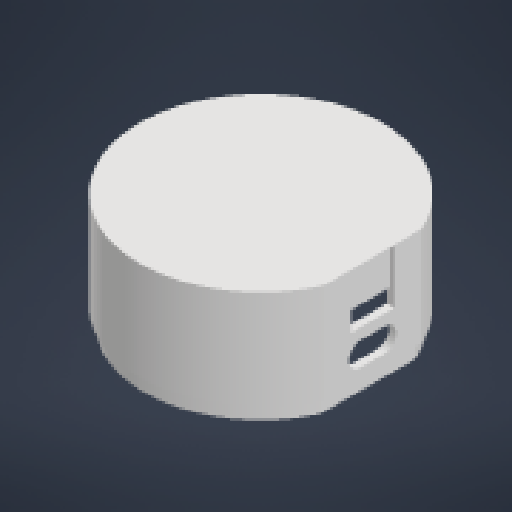
# Autodesk Inventor part: Boden
Saved by Autodesk Inventor 2026 (Build 300175000, 175)
## iProperties
Created: 2025-04-23
Part Number: Boden
Material: Generisch
Document SubType Name: Modeling
Designer: HTL
Density: 1 g/cm^3
Appearance: Vorgabe
Author: HTL
Autodesk Inventor part; units mm, degrees
ref_plane "YZ Plane" through (0, 0, 0) normal (1, 0, 0) x (0, 1, 0)
ref_plane "XZ Plane" through (0, 0, 0) normal (0, 1, 0) x (-1, 0, 0)
ref_plane "XY Plane" through (0, 0, 0) normal (0, 0, 1) x (1, 0, 0)
ref_plane "Arbeitsebene1" through (16.6353, -6.4369, 0) normal (0, 0, 1) x (1, 0, 0)
sketch "Skizze1" plane through (16.6353, -6.4369, 0) normal (0, 0, 1) x (1, 0, 0)
  circle A0 centre (-16.6375, -8.7) radius 1.3
  circle A1 centre (-16.6375, 8.7) radius 1.3
  circle A2 centre (23.3088, -8.7) radius 1.3
  circle A3 centre (23.3715, 8.7) radius 1.3
  point P0 (-16.6353, 6.4369)
  constraints: 4 centre point
extrude "Extrusion1" add sketch "Skizze1" along normal mid plane 4
ref_plane "Arbeitsebene3" through (16.6353, -6.4369, 0) normal (0, 0, 1) x (1, 0, 0)
sketch "Skizze11" plane through (16.6353, -6.4369, 0) normal (0, 0, 1) x (1, 0, 0)
  line L0 (19.6375, -11.7) -> (-19.6375, -11.7)
  line L1 (-19.6375, -11.7) -> (-19.6375, 11.7)
  line L2 (-20.6375, 12.7) -> (27.3715, 12.7)
  line L3 (-19.6375, 11.7) -> (-19.6375, -11.7)
  line L4 (-19.6375, -11.7) -> (26.3715, -11.7)
  line L5 (26.3715, -11.7) -> (26.3715, 11.7)
  line L6 (-19.6375, 11.7) -> (26.3715, 11.7)
  line L7 (-20.6375, -12.7) -> (27.3715, -12.7)
  line L8 (27.3715, -12.7) -> (27.3715, 12.7)
  line L9 (-20.6375, -12.7) -> (27.3715, -12.7)
  line L10 (27.3715, -12.7) -> (27.3715, 12.7)
  line L11 (27.3715, 12.7) -> (-20.6375, 12.7)
  line L12 (-20.6375, 12.7) -> (-20.6375, -12.7)
  point P0 (-16.6353, 6.4369)
  point P1 (19.6375, -11.7)
  constraints: 26 end point, 3 horizontal, 3 parallel, 3 perpendicular
sketch "Skizze12" plane through (16.6353, -6.4369, 2) normal (0, 0, 1) x (1, 0, 0)
  line L0 (20.6375, 12.7) -> (-20.6375, 12.7) projected
  line L1 (-20.6375, 12.7) -> (-20.6375, -12.7) projected
  line L2 (-20.6375, -12.7) -> (20.6375, -12.7) projected
  line L3 (20.6375, -12.7) -> (20.6375, 12.7) projected
  circle A0 centre (0, 0) radius 32
  line L4 (20.6375, 12.7) -> (29.3719, 12.7)
  line L5 (29.3719, -12.7) -> (20.6375, -12.7)
  line L6 (29.3719, -12.7) -> (29.3719, 12.7)
  point P0 (-16.6353, 6.4369)
  dimension "d20" = 64
  constraints: 6 end point, 2 point on circle, 1 centre point, 1 horizontal, 1 parallel, 1 perpendicular
  measures "d20" diameter of A0
extrude "Extrusion7" add sketch "Skizze12" along normal blind 2 contours L3 L2 L1 L0 | L4 L6 L5 L3 | L0 L1 L2 L5 A0 L4
sketch "Skizze13" plane through (16.6353, -6.4369, 2) normal (0, 0, -1) x (-1, 0, 0)
  arc A0 (-29.3719, -12.7) -> (-29.3719, 12.7) centre (0, 0) ccw projected
  line L0 (-29.3719, -12.7) -> (-29.3719, 12.7) projected
  arc A1 (-27.3719, -12.2792) -> (-27.3719, 12.2792) centre (0, 0) ccw
  line L1 (-27.3719, -12.2792) -> (-27.3719, 12.2792)
  point P0 (16.6353, 6.4369)
  dimension "d23" = 2
  constraints: 2 end point, 2 point on circle, 1 centre point, 1 other
  measures "d23" distance between parallel lines of L0 L1
extrude "Extrusion8" add sketch "Skizze13" along normal blind 24
sketch "Skizze14" plane through (16.6353, -6.4369, -22) normal (0, 0, -1) x (-1, 0, 0)
  line L0 (-27.3719, -12.2792) -> (-27.3719, 12.2792) projected
  arc A0 (-27.3719, -12.2792) -> (-27.3719, 12.2792) centre (0, 0) ccw projected
  line L1 (-28.1719, 12.4492) -> (-28.1719, -12.4492)
  arc A1 (-28.1719, -12.4492) -> (-28.1719, 12.4492) centre (0, 0) ccw
  point P0 (16.6353, 6.4369)
  dimension "d26" = 0.8
  constraints: 2 end point, 2 point on circle, 1 centre point, 1 other
  measures "d26" distance between parallel lines of L0 L1
extrude "Extrusion9" add sketch "Skizze14" along normal blind 4
sketch "Skizze18" plane through (46.0073, -19.1369, 4) normal (1, 0, 0) x (0, 0, -1)
  line L0 (18.8305, 15.87) -> (18.8305, 9.53) construction
  line L1 (18.8305, 15.87) -> (18.8305, 12.7)
  line L2 (20.4105, 15.87) -> (20.4105, 9.53) construction
  line L3 (18.8305, 9.53) -> (18.8305, 15.87)
  line L4 (18.8305, 15.87) -> (18.8305, 9.53) construction
  line L5 (20.4105, 15.87) -> (20.4105, 9.53) construction
  line L6 (21.9905, 15.87) -> (21.9905, 9.53)
  line L7 (18.8305, 9.53) -> (18.8305, 15.87)
  arc A0 (21.9905, 15.87) -> (18.8305, 15.87) centre (20.4105, 15.87) ccw
  arc A1 (18.8305, 9.53) -> (21.9905, 9.53) centre (20.4105, 9.53) ccw
  line L8 (23.4905, 9.53) -> (23.4905, 15.87)
  arc A2 (23.4905, 15.87) -> (17.3305, 15.87) centre (20.4105, 15.87) ccw
  line L9 (17.3305, 15.87) -> (17.3305, 9.53)
  arc A3 (17.3305, 9.53) -> (23.4905, 9.53) centre (20.4105, 9.53) ccw
  line L10 (26, 25.4) -> (0, 25.4) projected
  line L11 (0, 0) -> (26, 0) projected
  point P0 (4, 19.1369)
  point P1 (20.4105, 12.7)
  point P2 (18.8305, 12.7)
  point P3 (20.4105, 12.7)
  dimension "d75" = 1.5
  constraints: 28 end point, 8 point on circle, 4 centre point, 4 midpoint, 4 tangent, 3 parallel, 1 collinear, 1 vertical, 3 other
  measures "d75" distance between parallel lines of L6 L8
extrude "Extrusion10" cut sketch "Skizze18" against normal blind 4 contours A0 L6 A1 L3 L1 | A3 L9 A2 L8
sketch "Skizze19" plane through (46.0073, -19.1369, 4) normal (1, 0, 0) x (0, 0, -1)
  arc A0 (14.7505, 9.53) -> (22.9105, 9.53) centre (18.8305, 9.53) ccw projected
  line L0 (14.7505, 9.53) -> (14.7505, 15.87) projected
  arc A1 (22.9105, 15.87) -> (14.7505, 15.87) centre (18.8305, 15.87) ccw projected
  line L1 (0.5305, 7.35) -> (14.0305, 18.05) construction
  line L2 (0.5305, 18.05) -> (14.0305, 7.35) construction
  line L3 (14.3305, 7.05) -> (14.3305, 18.35)
  line L4 (14.3305, 18.35) -> (0.2305, 18.35)
  line L5 (0.2305, 18.35) -> (0.2305, 7.05)
  line L6 (0.2305, 7.05) -> (14.3305, 7.05)
  point P0 (4, 19.1369)
  dimension "d43" = 10.7
  dimension "d44" = 13.5
  constraints: 12 end point, 2 parallel, 1 perpendicular
  measures "d43" distance of L1.start L2.start
  measures "d44" distance of L2.start L1.end
extrude "Extrusion11" cut sketch "Skizze19" against normal blind 1.2
sketch "Skizze20" plane through (44.8073, -19.1369, 4) normal (1, 0, 0) x (0, 0, -1)
  line L0 (14.3305, 18.35) -> (14.3305, 7.05) projected
  line L1 (0.2305, 18.35) -> (14.3305, 18.35) projected
  line L2 (14.3305, 7.05) -> (0.2305, 7.05) projected
  line L3 (14.3305, 18.35) -> (10.3305, 18.35)
  line L4 (10.3305, 18.35) -> (10.3305, 7.05)
  line L5 (10.3305, 7.05) -> (14.3305, 7.05)
  line L6 (14.3305, 7.05) -> (14.3305, 18.35)
  point P0 (4, 19.1369)
  dimension "d49" = 4
  constraints: 8 end point, 2 parallel, 1 horizontal, 1 perpendicular, 1 point on line
  measures "d49" distance of L5.end L4.end
extrude "Extrusion12" cut sketch "Skizze20" against normal blind 1.2
extrude "Extrusion14" add sketch "Skizze11" along normal blind 2
